snowman cards_v2 (Autodesk Fusion 360 design; units mm, degrees)
Autodesk Fusion 360 part; units mm, degrees
sketch "snowman" plane through (0, 0, 0) normal (0, 0, 1) x (1, 0, 0)
  line L0 (54.983, 94.7626) -> (55.1205, 94.7626)
  line L1 (55.1205, 122.9836) -> (38.9981, 122.9836)
  line L2 (38.9981, 122.9836) -> (38.9981, 100.7922)
  arc A0 (50.4427, 75.848) -> (54.983, 94.7626) centre (47.5314, 86.549) ccw
  arc A1 (40.2055, 94.8749) -> (44.4581, 75.8933) centre (47.5314, 86.549) ccw
  circle A2 centre (41.4945, 90.3986) radius 2.0028
  circle A3 centre (52.4993, 90.3475) radius 2.0028
  line L3 (47.338, 61.0384) -> (44.7084, 24.9416) construction
  line L4 (14.9544, 56.2681) -> (10.1054, 54.2248)
  line L5 (15.0769, 56.0048) -> (10.1992, 53.9983)
  line L6 (32.4801, 63.1415) -> (14.9544, 56.2681)
  line L7 (31.3312, 62.6913) -> (15.0769, 56.0048)
  spline S0 degree 5 poles (41.4945, 83.5543) (41.6944, 83.3364) (42.0935, 82.9196) (42.6899, 82.3512) (43.4803, 81.7088) (44.46, 81.1114) (45.4306, 80.7382) (46.3913, 80.6082) (47.3416, 80.7324) (48.282, 81.102) (49.2131, 81.6989) (49.9513, 82.3436) (50.5013, 82.9153) (50.8664, 83.3349) (51.0485, 83.5543) knots 0 0 0 0 0 0 0.1 0.2 0.3 0.4 0.5 0.6 0.7 0.8 0.9 1 1 1 1 1 1
  circle A4 centre (47.5314, 86.549) radius 1.5
  circle A5 centre (46.8803, 68.1808) radius 2.1619
  circle A6 centre (46.8803, 42.3308) radius 2.1619
  line L8 (47.338, 35.1884) -> (44.7084, -0.9084) construction
  circle A7 centre (46.8803, 16.4808) radius 2.1619
  line L9 (47.338, 9.3384) -> (44.7084, -26.7584) construction
  arc A8 (33.8102, 98.018) -> (40.2055, 94.8749) centre (47.7731, 118.3505) ccw
  arc A9 (54.983, 94.7626) -> (61.0922, 97.5906) centre (47.7731, 118.3505) ccw
  line L10 (62.2248, 59.1511) -> (79.5719, 53.1868)
  line L11 (33.581, 67.34) -> (11.7153, 58.7645)
  line L12 (11.7153, 58.7645) -> (7.3408, 58.7645)
  line L13 (3.6772, 59.3481) -> (3.6772, 59.2727)
  arc A10 (44.4581, 75.8933) -> (33.581, 67.34) centre (47.338, 61.0384) ccw
  arc A11 (53.973, 47.579) -> (62.2248, 59.1511) centre (47.338, 61.0384) ccw
  arc A12 (62.1108, 64.3138) -> (50.4427, 75.848) centre (47.338, 61.0384) ccw
  line L14 (55.1205, 94.7626) -> (55.1205, 94.805)
  line L15 (55.1205, 99.7518) -> (55.1205, 122.9836)
  spline S1 degree 5 poles (61.0922, 97.5906) (60.8581, 97.7021) (60.3893, 97.9223) (59.6844, 98.2439) (58.741, 98.6539) (57.5531, 99.12) (56.5913, 99.4322) (55.8602, 99.6151) (55.3679, 99.7107) (55.1205, 99.7518) knots 0 0 0 0 0 0 0.2 0.4 0.6 0.8 1 1 1 1 1 1
  line L16 (55.6951, 99.6562) -> (54.5459, 99.8474)
  spline S2 degree 5 poles (38.9981, 100.7922) (38.7345, 100.7613) (38.2249, 100.6704) (37.5136, 100.4468) (36.6557, 100.0029) (35.6758, 99.3199) (34.9259, 98.7598) (34.3679, 98.3715) (33.9961, 98.1325) (33.8102, 98.018) knots 0 0 0 0 0 0 0.2 0.4 0.6 0.8 1 1 1 1 1 1
  line L17 (39.7359, 100.8787) -> (38.2604, 100.7057)
  line L18 (34.3477, 98.3493) -> (33.2727, 97.6868)
  line L19 (62.1108, 64.3138) -> (80.423, 57.5844)
  spline S3 degree 5 poles (80.423, 57.5844) (80.7574, 57.8719) (81.4136, 58.4121) (82.3598, 59.1183) (83.5449, 59.8513) (84.8978, 60.4207) (86.12, 60.6498) (87.208, 60.5542) (88.1574, 60.1635) (88.9622, 59.5241) (89.6147, 58.7051) (90.1092, 57.7865) (90.4463, 56.8432) (90.6365, 55.9314) (90.7059, 55.0725) (90.6974, 54.2431) (90.6518, 53.402) (90.5916, 52.5127) (90.5036, 51.5666) (90.3213, 50.6074) (89.9565, 49.709) (89.3343, 48.9503) (88.423, 48.3948) (87.277, 48.0608) (86.0316, 47.921) (84.8475, 47.9301) (83.8672, 48.0458) (83.1716, 48.2501) (82.7229, 48.5772) (82.3638, 49.1135) (81.8822, 49.9685) (81.223, 50.9953) (80.4965, 51.9968) (79.8989, 52.7722) (79.5719, 53.1868) knots 0 0 0 0 0 0 0.033333 0.066667 0.1 0.133333 0.166667 0.2 0.233333 0.266667 0.3 0.333333 0.366667 0.4 0.433333 0.466667 0.5 0.533333 0.566667 0.6 0.633333 0.666667 0.7 0.733333 0.766667 0.8 0.833333 0.866667 0.9 0.933333 0.966667 1 1 1 1 1 1
  line L20 (83.5315, 48.1676) -> (75.6122, 58.206)
  spline S4 degree 5 poles (10.1992, 53.9983) (10.3009, 53.6952) (10.48, 53.1083) (10.6755, 52.2856) (10.7895, 51.3046) (10.6882, 50.2732) (10.3484, 49.4383) (9.7841, 48.8012) (9.021, 48.3619) (8.102, 48.1178) (7.0835, 48.0641) (6.029, 48.1933) (5.0031, 48.4953) (4.0663, 48.9576) (3.2683, 49.5646) (2.6456, 50.2976) (2.2225, 51.1346) (2.0101, 52.0504) (2.0069, 53.0157) (2.1968, 53.9972) (2.5533, 54.9589) (3.0441, 55.8652) (3.6359, 56.6836) (4.2982, 57.3871) (5.0092, 57.9575) (5.7559, 58.3854) (6.3766, 58.6105) (6.854, 58.7131) (7.1777, 58.7523) (7.3408, 58.7645) knots 0 0 0 0 0 0 0.04 0.08 0.12 0.16 0.2 0.24 0.28 0.32 0.36 0.4 0.44 0.48 0.52 0.56 0.6 0.64 0.68 0.72 0.76 0.8 0.84 0.88 0.92 0.96 1 1 1 1 1 1
  arc A13 (38.8223, 48.6827) -> (46.6987, 0.5628) centre (44.7084, 24.9416) ccw
  arc A14 (44.8097, 0.4819) -> (53.973, 47.579) centre (44.7084, 24.9416) ccw
  arc A15 (46.6987, 0.5628) -> (53.973, 47.579) centre (44.7084, 24.9416) ccw
  arc A16 (38.8223, 48.6827) -> (44.8097, 0.4819) centre (44.7084, 24.9416) ccw
  arc A17 (32.4801, 63.1415) -> (38.8223, 48.6827) centre (47.338, 61.0384) ccw
  point P0 (46.4404, 80.6718)
  point P1 (88.2593, 60.0171)
  point P2 (90.5817, 56.098)
  point P3 (90.5817, 52.4693)
  point P4 (88.8399, 48.6954)
  point P5 (83.5315, 48.1676)
  point P6 (9.5237, 48.6954)
  point P7 (4.6528, 48.6954)
  point P8 (2.0401, 52.3241)
  point P9 (3.9271, 56.9689)
  dimension "d12" = 3
  dimension "d15" = 0
  dimension "d16" = -51.7
  constraint concentric A10 A11
  constraint horizontal L0
  constraint vertical L14
  constraint horizontal L1
  constraint vertical L2
  constraint coincident A1.start A0
  constraint coincident L0.start A8
  constraint concentric A0 A1
  constraint coincident L3.start A10.centre
  constraint coincident L3.end A13.centre
  constraint concentric A0 A4
  constraint concentric A8 A9
  constraint parallel L6 L11
  constraint horizontal L12
  constraint perpendicular L12 L13
  constraint concentric A10 A17
  constraint concentric A11 A12
  constraint coincident A9 L14.end
  constraint collinear L14 L15
  constraint midpoint L15.start L16
  constraint midpoint L2.end L17
  constraint midpoint A8.start L18
  constraint midpoint L10.end L20
  constraint coincident P5 L20.start
  constraint coincident L9 A13.end
  constraint concentric A13 A15
  constraint coincident L8 A14.start
  constraint concentric A14 A15
  constraint concentric A15 A16
  measures "d12" diameter of A4
extrude "Extrude1" add sketch "snowman" along normal blind 0.5 contours L1 L2 A0 A1 L5 L6 L7 A8 A9 L10 L11 L12 A10 A11 A12 L15 S1 S2 L19 S3 L20 S4 A13 A14 A15 A16 A17 | S3 L20
